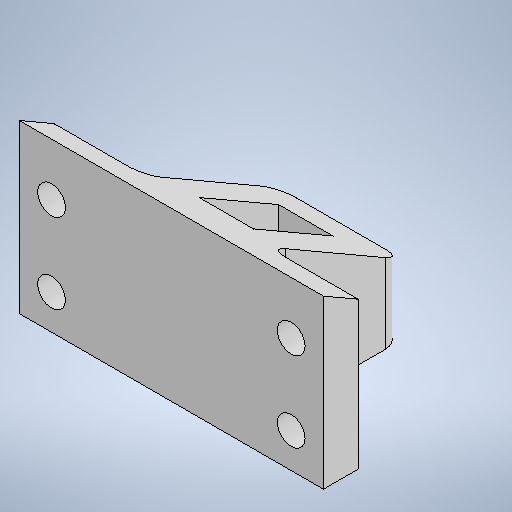
# Autodesk Inventor part: TopMotorMount
Saved by Autodesk Inventor 2026 (Build 300175050, 175E)
## iProperties
Created: 2025-12-26
Part Number: TopMotorMount
Material: Generic
Document SubType Name: Modeling
Designer: Nicholas M
Density: 1 g/cm^3
Appearance: Default
Author: Nicholas M
Autodesk Inventor part; units mm, degrees
ref_plane "YZ Plane" through (0, 0, 0) normal (1, 0, 0) x (0, 1, 0)
ref_plane "XZ Plane" through (0, 0, 0) normal (0, 1, 0) x (-1, 0, 0)
ref_plane "XY Plane" through (0, 0, 0) normal (0, 0, 1) x (1, 0, 0)
sketch "Sketch1" plane through (0, 0, 0) normal (0, 0, 1) x (1, 0, 0)
  line L0 (0, 0) -> (6.25, 0)
  line L1 (6.25, 0) -> (6.25, 8)
  line L2 (6.25, 8) -> (0, 8)
  line L3 (0, 8) -> (0, 0)
  line L4 (6.25, 0) -> (10.25, 0)
  line L5 (10.25, 0) -> (10.25, 8)
  line L6 (10.25, 8) -> (6.25, 8)
  line L7 (6.25, 8) -> (6.25, 0)
  line L8 (0, 0) -> (-4, 0)
  line L9 (-4, 0) -> (-4, 8)
  line L10 (-4, 8) -> (0, 8)
  line L11 (0, 8) -> (0, 0)
  point P0 (6.25, 4)
  point P1 (3.125, 8)
  dimension "d0" = 6.25
  dimension "d1" = 8
  dimension "d3" = 4
  constraints: 24 end point, 6 parallel, 3 horizontal, 3 perpendicular, 2 collinear, 2 midpoint, 1 point on line
  measures "d0" distance of L2.end L1.end
  measures "d1" distance of L0.end L1.end
  measures "d3" distance of L6.end L5.end
extrude "Extrusion1" add sketch "Sketch1" along normal blind 9.15 contours L8 L9 L10 L3 | L1 L6 L5 L4
extrude "Extrusion2" add sketch "Sketch1" against normal blind 4
sketch "Sketch2" plane through (10.25, 0, 9.15) normal (1, 0, 0) x (0, 0, -1)
  line L0 (9.15, 0) -> (9.15, 8) projected
  line L1 (9.15, 8) -> (0, 8) projected
  line L2 (0, 0) -> (0, 8) projected
  line L3 (9.15, 0) -> (0, 0) projected
  circle A0 centre (4.575, 4) radius 1.6
  line L4 (0, 0) -> (0, 8) projected
  point P0 (0, 4)
  point P1 (4.575, 8)
  dimension "d8" = 3.2
  constraints: 2 midpoint, 1 centre point, 1 horizontal alignment, 1 vertical alignment
  measures "d8" diameter of A0
extrude "Extrusion3" cut sketch "Sketch2" against normal through all contours A0
extrude "Extrusion4" add sketch "Sketch1" along normal blind 4 from surface at 9.15
sketch "Sketch3" plane through (10.25, 0, -4) normal (1, 0, 0) x (0, 0, -1)
  line L0 (-17.15, 17.9016) -> (-17.15, -9.9016)
  line L1 (-17.15, -9.9016) -> (0, 0)
  line L2 (0, 0) -> (0, 8)
  line L3 (0, 8) -> (-17.15, 17.9016)
  line L4 (-17.15, 8) -> (-17.15, 0) projected
  circle A0 centre (-8.575, 4) radius 1.6 projected
  line L5 (0, 0) -> (-17.15, 0) projected
  line L6 (-19.475, 19.2439) -> (-19.475, -11.2439)
  line L7 (-17.15, 17.9016) -> (-19.475, 19.2439)
  line L8 (-19.475, -11.2439) -> (-17.15, -9.9016)
  line L9 (-17.15, 0) -> (-19.475, 0)
  point P0 (-4, 0)
  dimension "d13" = 60
  dimension "d20" = 2.325
  constraints: 16 end point, 3 collinear, 2 vertical, 1 coincident, 1 equal length, 1 horizontal, 1 parallel, 1 point on line
  measures "d13" angle of L1 L0
  measures "d20" distance between parallel lines of L0 L6
sketch "Sketch4" plane through (-4, 8, -4) normal (0, 1, 0) x (1, 0, 0)
  line L0 (4, -13.15) -> (10.25, -13.15) projected
  line L1 (10.25, -4) -> (10.25, -13.15) projected
  line L2 (4, -4) -> (4, -13.15) projected
  line L3 (10.25, -4) -> (4, -4) projected
extrude "Extrusion5" add sketch "Sketch3" against normal up to surface (14.25 mm away) contours L3 L2 L5 L0 | L0 L9 L6 L7
extrude "Extrusion6" cut sketch "Sketch4" along normal through all both and the other way through all
sketch "Sketch5" plane through (10.25, 0, 15.475) normal (1, 0, 0) x (0, 0, -1)
  circle A0 centre (10.9, 4) radius 1.6 projected
  line L0 (19.475, 8) -> (0, 19.2439) projected
  line L1 (0, 19.2439) -> (0, 0) projected
  line L2 (19.475, 0) -> (0, 0) projected
  line L3 (19.475, 8) -> (19.475, 0) projected
  line L4 (4, 16.9345) -> (4, 0)
  point P0 (15.475, 0)
  dimension "d21" = 4
  constraints: 2 end point, 2 point on line, 1 vertical
  measures "d21" distance between parallel lines of L1 L4
extrude "Extrusion7" add sketch "Sketch5" along normal blind 10.375 and the other way blind 24.625 contours L4 L2 L1 L0
sketch "Sketch6" plane through (10.25, 0, 11.475) normal (0, 0, -1) x (-1, 0, 0)
  circle A0 centre (-6.6625, 13.2) radius 1.6
  line L0 (-10.375, 0) -> (-10.375, 16.9345) projected
  line L1 (0, 16.9345) -> (-10.375, 16.9345) projected
  circle A1 centre (20.9125, 13.2) radius 1.6
  circle A2 centre (20.9125, 4) radius 1.6
  circle A3 centre (-6.6625, 4) radius 1.6
  line L2 (0, 0) -> (-10.375, 0) projected
  line L3 (24.625, 16.9345) -> (24.625, 0) projected
  point P0 (10.25, 0)
  dimension "d26" = 3.2
  dimension "d27" = 3.7125
  dimension "d29" = 4
  dimension "d30" = 3.7125
  dimension "d34" = 6
  constraints: 4 centre point, 3 equal radius, 2 horizontal alignment, 2 vertical alignment
  measures "d26" diameter of A0
  measures "d27" distance from line of L0 A0.centre
  measures "d29" distance from line of L2 A3.centre
  measures "d30" distance from line of L3 A1.centre
extrude "Extrusion8" cut sketch "Sketch6" against normal through all
fillet "Fillet1" radius 2 4 edges at (10.25, 8.4672, 11.475) (-4, 8.4672, 11.475) (10.25, 4, -4) (-4, 4, -4)
body "Solid1"
